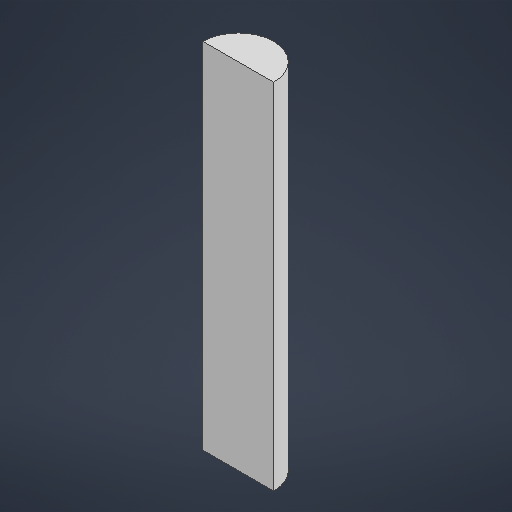
# Autodesk Inventor part: モーターの釘
Saved by Autodesk Inventor 2026 (Build 300175000, 175)
## iProperties
Created: 2025-10-27
Part Number: モーターの釘
Material: 一般
Document SubType Name: Modeling
Designer: masak
Density: 1 g/cm^3
Appearance: 既定
Author: masak
Autodesk Inventor part; units mm, degrees
ref_plane "YZ Plane" through (0, 0, 0) normal (1, 0, 0) x (0, 1, 0)
ref_plane "XZ Plane" through (0, 0, 0) normal (0, 1, 0) x (-1, 0, 0)
ref_plane "XY Plane" through (0, 0, 0) normal (0, 0, 1) x (1, 0, 0)
sketch "スケッチ1" plane through (0, 0, 0) normal (0, 1, 0) x (-1, 0, 0)
  circle A0 centre (0, 0) radius 1.5
  line L0 (1.5, 0) -> (-1.5, 0)
  dimension "d0" = 3
  constraints: 2 end point, 2 point on circle, 1 centre point, 1 coincident, 1 horizontal
  measures "d0" diameter of A0
extrude "押し出し1" add sketch "スケッチ1" along normal blind 15 contours A0 L0 picked at (-0.4427, -0.2324)
